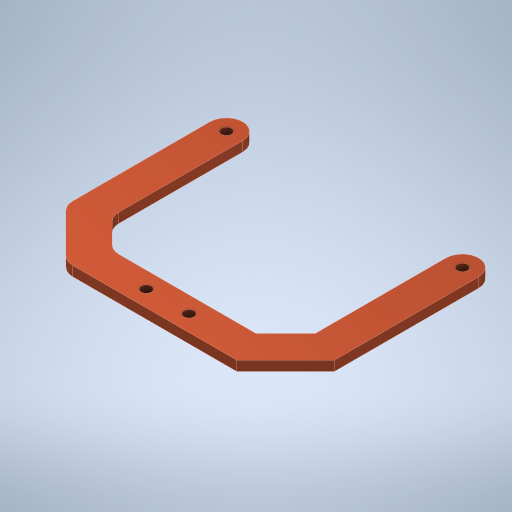
# Autodesk Inventor part: Claw4
Saved by Autodesk Inventor 2023.2 (Build 272271030, 271C)
## iProperties
Created: 2022-11-29
Part Number: Claw4
Material: Copper, Cast
Document SubType Name: Modeling
Designer: kakik
Density: 8.94 g/cm^3
Appearance: Copper - Satin
Author: kakik
Autodesk Inventor part; units mm, degrees
ref_plane "YZ Plane" through (0, 0, 0) normal (1, 0, 0) x (0, 1, 0)
ref_plane "XZ Plane" through (0, 0, 0) normal (0, 1, 0) x (-1, 0, 0)
ref_plane "XY Plane" through (0, 0, 0) normal (0, 0, 1) x (1, 0, 0)
sketch "Sketch3" plane through (0, 0, 0) normal (0, 1, 0) x (-1, 0, 0)
  line L0 (0, 0) -> (22, 0)
  line L1 (31.1421, -9.1421) -> (31.1421, -49.1421)
  line L2 (41.1421, -49.1421) -> (41.1421, -5)
  line L3 (0, 10) -> (0, 0)
  line L4 (26.1421, 10) -> (41.1421, -5)
  line L5 (31.1421, -9.1421) -> (22, 0)
  line L6 (26.1421, 10) -> (0, 10)
  line L7 (22, 0) -> (0, 0)
  line L8 (31.1421, -9.1421) -> (31.1421, -49.1421)
  line L9 (41.1421, -49.1421) -> (41.1421, -5)
  line L10 (22, 0) -> (0, 0)
  arc A0 (31.1421, -49.1421) -> (41.1421, -49.1421) centre (36.1421, -49.1421) ccw
  circle A1 centre (0, -30) radius 30
  point P0 (31.1421, -29.1421)
  dimension "d51" = 10
  dimension "d56" = 10
  dimension "d57" = 15
  dimension "d58" = 15
  dimension "d59" = 5
  dimension "d60" = 22
  dimension "d61" = 40
  dimension "d64" = 10
  dimension "d65" = 10
  dimension "d66" = 60
  dimension "d67" = 30
  constraints: 22 end point, 3 perpendicular, 2 centre point, 2 point on circle, 1 collinear, 1 horizontal, 1 horizontal alignment, 1 midpoint, 1 parallel, 1 tangent
  measures "d51" distance of L3.start L0.start
  measures "d56" distance between parallel lines of L5 L4
  measures "d57" horizontal distance of L4.start L2.end
  measures "d58" horizontal distance of L4.start L2.end
  measures "d59" radius of A0
  measures "d60" distance of L0.start L0.end
  measures "d61" distance of L1.start L1.end
  measures "d64" distance from line of point (31.142, -29.142) L2
  measures "d65" vertical distance of L4.start L0.end
  measures "d66" diameter of A1
  measures "d67" distance of L0.start A1.centre
extrude "Extrusion2" add sketch "Sketch3" along normal blind 3 contours L3 L6 L4 L2 A0 L1 L5 L0
sketch "Sketch4" plane through (0, 3, 0) normal (0, 1, 0) x (1, 0, 0)
  line L0 (0, -10) -> (0, 0) projected
  arc A0 (-31.1421, 49.1421) -> (-41.1421, 49.1421) centre (-36.1421, 49.1421) ccw projected
  point P0 (-6.55, -5)
  point P1 (0, -5)
  point P2 (-36.1421, 54.1421)
  dimension "d77" = 6.55
  constraints: 2 horizontal alignment, 1 midpoint, 1 point on circle, 1 vertical alignment
  measures "d77" distance from line of L0 point (-6.55, -5)
hole "Hole2" at (-6.55, 3, 5) at (-36.1421, 3, -49.1421) direction (0, -1, 0) diameter 3.2 end through all clearance for "Countersunk Flat Head Screw DIN EN ISO 2009" size "M3" standard "DIN"
fillet "Fillet1" radius 5 4 edges at (-26.1421, 1.5, 10) (-41.1421, 1.5, -5) (-31.1421, 1.5, -9.1421) (-22, 1.5, 0)
mirror "Mirror3" about plane through (0, 0, 10) normal (1, 0, 0) of "Extrusion2", "Hole2"
body "Solid2"
